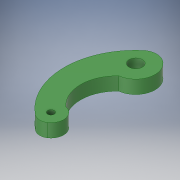
# Autodesk Inventor part: МД.001.1004 - Толкатель
Saved by Autodesk Inventor 2019 (Build 230136000, 136)
## iProperties
Created: 2020-01-02
Part Number: МД.001.1004 - Толкатель
Material: Пластик АБС
Document SubType Name: Modeling
Designer: Петров Иван
Density: 1.06 g/cm^3
Appearance: Гладкий — темный травянисто-зеленый
Author: Петров Иван
Autodesk Inventor part; units mm, degrees
ref_plane "YZ Plane" through (0, 0, 0) normal (1, 0, 0) x (0, 1, 0)
ref_plane "XZ Plane" through (0, 0, 0) normal (0, 1, 0) x (-1, 0, 0)
ref_plane "XY Plane" through (0, 0, 0) normal (0, 0, 1) x (1, 0, 0)
sketch "Эскиз1" plane through (0, 0, 0) normal (0, 1, 0) x (-1, 0, 0)
  circle A0 centre (0, 0) radius 1
  line L0 (0, 0) -> (0, -25.47)
  circle A1 centre (0, -25.47) radius 2
  circle A2 centre (0, 0) radius 2
  arc A3 (4, -25.47) -> (0, -29.47) centre (0, -25.47) ccw
  arc A4 (0, -29.47) -> (0, 2) centre (-11.735, -13.735) ccw
  arc A5 (0, -21.47) -> (0, -2) centre (-8.0108, -11.735) ccw
  dimension "d0" = 2
  dimension "d1" = 25.47
  dimension "d2" = 4
  dimension "d3" = 4
  dimension "d4" = 8
  constraints: 10 point on circle, 6 centre point, 4 coincident, 2 end point, 2 point on line, 1 vertical
  measures "d0" diameter of A0
  measures "d1" distance of L0.start L0.end
  measures "d2" diameter of A1
  measures "d3" diameter of A2
  measures "d4" diameter of A3
extrude "Выдавливание1" add sketch "Эскиз1" along normal blind 4 contours A2 A4 | A2 A4 A3 A5 | A3 A4 picked at (0.2552, 1.4877)
fillet "Сопряжение1" radius 2.75 1 edges at (0, 2, -29.47)
fillet "Сопряжение2" radius 1.4 1 edges at (0, 2, 2)
thicken "Толщина1" operation add thickness 1.8 both sides no extend neighbours yes toward (-0.7073284, 0, -0.7068851) faces at (-2.1492, 2.6667, -27.6105) (0.8001, 2.6667, -29.2545) (3.5299, 2.6667, -23.5885) (-0.6934, 2.6667, -20.8553) (1.2582, 1.3333, 1.5546) (0.1882, 1.3333, 1.8857)
